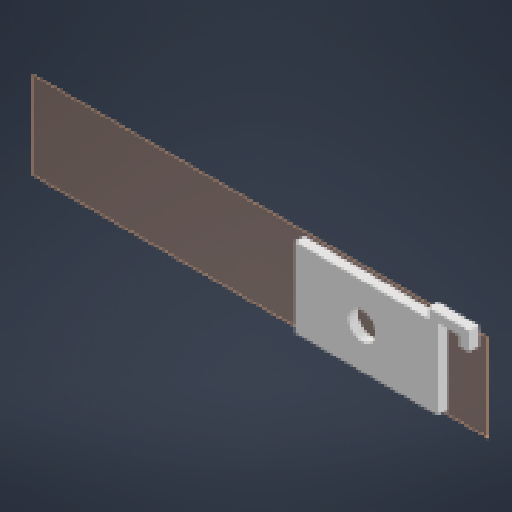
# Autodesk Inventor part: Button Bracket 2
Saved by Autodesk Inventor 2025.2 (Build 292293000, 293)
## iProperties
Created: 2024-11-20
Part Number: Button Bracket 2
Material: Generic
Document SubType Name: Modeling
Designer: JL
Density: 1 g/cm^3
Appearance: Default
Author: JL
Autodesk Inventor part; units mm, degrees
ref_plane "YZ Plane" through (0, 0, 0) normal (1, 0, 0) x (0, 1, 0)
ref_plane "XZ Plane" through (0, 0, 0) normal (0, 1, 0) x (-1, 0, 0)
ref_plane "XY Plane" through (0, 0, 0) normal (0, 0, 1) x (1, 0, 0)
ref_plane "Work Plane1" through (0, 0, 0) normal (0, 0, 1) x (1, 0, 0)
sketch "Sketch1" plane through (0, 0, 0) normal (0, 0, 1) x (1, 0, 0)
  circle A0 centre (103.8623, 15.35) radius 2.15 construction
  circle A1 centre (103.8623, -15.35) radius 2.15 construction
  line L0 (-103.8623, 20.35) -> (-103.8623, -20.35) construction
  line L1 (108.8623, -20.35) -> (-103.8623, -20.35) construction
  line L2 (108.8623, 20.35) -> (108.8623, -20.35) construction
  line L3 (-103.8623, 20.35) -> (108.8623, 20.35) construction
  circle A2 centre (59.3407, 0) radius 6.5 construction
  circle A3 centre (59.3407, 0) radius 7
  circle A4 centre (59.3407, 0) radius 24.5216 construction
  line L4 (34.8192, 0) -> (24.8192, 0) construction
  line L5 (24.8192, -20.35) -> (24.8192, 20.35)
  line L6 (24.8192, 20.35) -> (98.3623, 20.35)
  line L7 (98.8623, -20.35) -> (98.8623, 20.35) construction
  line L8 (98.3623, -20.35) -> (24.8192, -20.35)
  line L9 (95.8623, -23.35) -> (95.8623, 9.65) projected
  line L10 (95.3623, -20.35) -> (24.8192, -20.35)
  line L11 (98.8623, 9.65) -> (95.8623, 9.65) projected
  line L12 (98.8623, 20.35) -> (98.8623, -20.35) projected
  line L13 (98.3623, 10.15) -> (95.3623, 10.15)
  line L14 (95.3623, 10.15) -> (95.3623, -23.3504)
  line L15 (98.3623, 10.15) -> (98.3623, 20.35)
  point P0 (0, 0)
  point P1 (95.3623, -20.35)
  dimension "d0" = 0.5
  dimension "d1" = 10
  dimension "d15" = 0.5
  dimension "d16" = 0.5
  dimension "d17" = 0.5
  constraints: 16 end point, 4 perpendicular, 3 point on line, 2 horizontal, 1 centre point, 1 horizontal alignment, 1 midpoint, 1 parallel, 1 other
  measures "d0" radial gap between concentric circles of A2 A3
  measures "d1" distance of L4.start L4.end
  measures "d15" distance between parallel lines of L11 L13
  measures "d16" distance between parallel lines of L7 L15
  measures "d17" distance between parallel lines of L9 L14
extrude "Extrusion1" add sketch "Sketch1" along normal blind 5
sketch "Sketch2" plane through (24.8192, -20.35, 0) normal (-1, 0, 0) x (0, 0, 1)
  line L0 (80.8, 35.7) -> (75.8, 35.7) construction
  line L1 (80.8, 45.7) -> (80.8, 35.7) construction
  line L2 (51.1, 45.7) -> (80.8, 45.7) construction
  line L3 (51.1, -4.2229) -> (51.1, 45.7) construction
  line L4 (26.6, -4.2229) -> (51.1, -4.2229) construction
  line L5 (26.6, -16.2229) -> (26.6, -4.2229) construction
  line L6 (65.2, -16.2229) -> (26.6, -16.2229) construction
  line L7 (65.2, 40.7) -> (65.2, -16.2229) construction
  line L8 (75.8, 40.7) -> (65.2, 40.7) construction
  line L9 (75.8, 35.7) -> (75.8, 40.7) construction
  line L10 (38.6, -16.2229) -> (0, -16.2229)
  line L11 (0, -16.2229) -> (0, -4.2229)
  line L12 (5, -4.2229) -> (38.6, -4.2229)
  line L13 (38.6, -4.2229) -> (38.6, -16.2229)
  line L14 (38.6, -10.2229) -> (26.6, -10.2229) construction
  line L15 (0, 40.7) -> (0, 0) construction
  line L16 (0, 0) -> (5, 0) construction
  line L17 (5, 40.7) -> (5, 0) construction
  line L18 (0, 40.7) -> (5, 40.7) construction
  line L19 (5, 5) -> (0, 5)
  line L20 (0, -4.2229) -> (0, 5)
  line L21 (5, 5) -> (5, -4.2229)
  point P0 (0, 20.35)
  dimension "d11" = 5
  constraints: 16 end point, 4 perpendicular, 3 collinear, 3 point on line, 2 midpoint, 2 parallel, 1 horizontal
  measures "d11" distance between parallel lines of L16 L19
extrude "Extrusion2" add sketch "Sketch2" against normal blind 5
equation "\"d15\" = d0"
equation "\"d16\" = d0"
equation "\"d17\" = d0"
equation "\"d9\" = d2"
equation "\"d11\" = d2"
equation "\"d12\" = d2"
equation "\"d2\" = 5"
body "Solid1"
